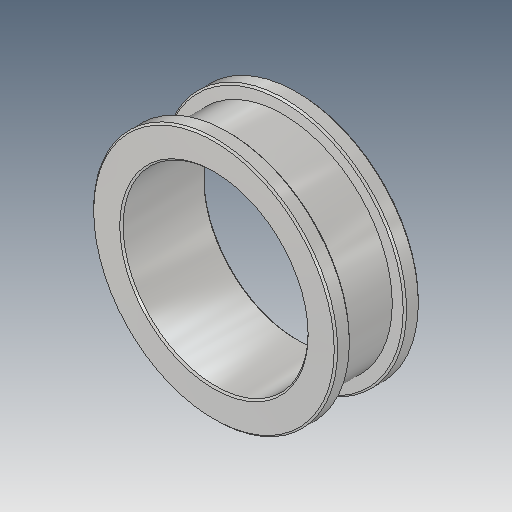
# Autodesk Inventor part: roller
Saved by Autodesk Inventor 2019 (Build 230136000, 136)
## iProperties
Created: 2018-11-16
Part Number: roller
Material: Aluminum 3004-H38
Document SubType Name: Modeling
Designer: LillaHunden
Density: 2.71043 g/cm^3
Appearance: Aluminum - Polished
Mass: 0.665565 g
Surface Area: 5.75714 cm^2
Volume: 0.245557 cm^3
Author: LillaHunden
Autodesk Inventor part; units mm, degrees
ref_plane "YZ Plane" through (0, 0, 0) normal (1, 0, 0) x (0, 1, 0)
ref_plane "XZ Plane" through (0, 0, 0) normal (0, 1, 0) x (-1, 0, 0)
ref_plane "XY Plane" through (0, 0, 0) normal (0, 0, 1) x (1, 0, 0)
sketch "Sketch1" plane through (0, 0, 0) normal (0, 0, 1) x (1, 0, 0)
  circle A0 centre (0, 0) radius 7.25
  dimension "d0" = 14.5
  constraints: 1 centre point, 1 coincident
  measures "d0" diameter of A0
extrude "Extrusion1" add sketch "Sketch1" along normal blind 5
sketch "Sketch2" plane through (0, 0, 5) normal (0, 0, 1) x (1, 0, 0)
  circle A0 centre (0, 0) radius 5.5
  dimension "d3" = 11
  constraints: 1 centre point, 1 coincident
  measures "d3" diameter of A0
extrude "Extrusion2" cut sketch "Sketch2" against normal through all
ref_plane "Work Plane1" through (0, 0, 2.5) normal (0, 0, 1) x (1, 0, 0)
sketch "Sketch3" plane through (0, 0, 2.5) normal (0, 0, 1) x (1, 0, 0)
  circle A0 centre (0, 0) radius 5.5 projected
  circle A1 centre (0, 0) radius 6.5
  circle A2 centre (0, 0) radius 7.25 projected
  dimension "d6" = 13
  constraints: 1 centre point, 1 coincident
  measures "d6" diameter of A1
extrude "Extrusion3" cut sketch "Sketch3" along normal mid plane 3.2 contours A2
chamfer "Chamfer1" distance 0.1 angle 45 6 edges at (-7.25, 0, 4.1) (-7.25, 0, 0.9) (-7.25, 0, 0) (-7.25, 0, 5) (-5.5, 0, 0) (-5.5, 0, 5)
body "Solid1"
